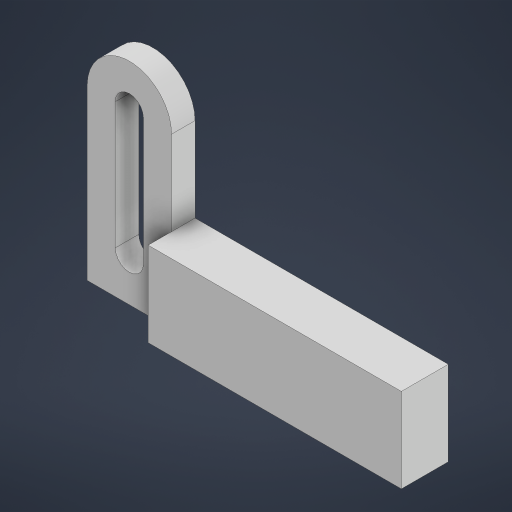
# Autodesk Inventor part: Slider2
Saved by Autodesk Inventor 2024 (Build 280153000, 153)
## iProperties
Created: 2024-02-06
Part Number: Slider2
Material: Generic
Document SubType Name: Modeling
Designer: calvi
Density: 1 g/cm^3
Appearance: Default
Author: calvi
Autodesk Inventor part; units mm, degrees
ref_plane "YZ Plane" through (0, 0, 0) normal (1, 0, 0) x (0, 1, 0)
ref_plane "XZ Plane" through (0, 0, 0) normal (0, 1, 0) x (-1, 0, 0)
ref_plane "XY Plane" through (0, 0, 0) normal (0, 0, 1) x (1, 0, 0)
sketch "Sketch1" plane through (0, 0, 0) normal (0, 0, 1) x (1, 0, 0)
  line L0 (0, 0) -> (22.86, 0)
  line L1 (22.86, 0) -> (22.86, 91.44)
  line L2 (22.86, 91.44) -> (0, 91.44)
  line L3 (0, 91.44) -> (0, 0)
  line L4 (22.86, 57.15) -> (91.44, 57.15)
  line L5 (91.44, 57.15) -> (91.44, 34.29)
  line L6 (91.44, 34.29) -> (22.86, 34.29)
  line L7 (22.86, 34.29) -> (22.86, 57.15)
  line L8 (11.43, 80.01) -> (11.43, 11.43) construction
  line L9 (7.62, 80.01) -> (7.62, 11.43)
  line L10 (15.24, 11.43) -> (15.24, 80.01)
  arc A0 (15.24, 80.01) -> (7.62, 80.01) centre (11.43, 80.01) ccw
  arc A1 (7.62, 11.43) -> (15.24, 11.43) centre (11.43, 11.43) ccw
  arc A2 (22.86, 80.01) -> (0, 80.01) centre (11.43, 80.01) ccw
  arc A3 (0, 11.43) -> (22.86, 11.43) centre (11.43, 11.43) ccw
  point P0 (11.43, 45.72)
  point P1 (-17.5605, -7.6237)
  dimension "d0" = 22.86
  dimension "d1" = 91.44
  dimension "d2" = 68.58
  dimension "d3" = 22.86
  dimension "d4" = 34.29
  dimension "d5" = 68.58
  dimension "d6" = 7.62
  dimension "d7" = 11.43
  dimension "d8" = 11.43
  dimension "d9" = 0
  dimension "d10" = 0
  constraints: 24 end point, 8 point on circle, 6 tangent, 5 parallel, 5 point on line, 4 centre point, 2 coincident, 2 horizontal, 2 perpendicular, 1 midpoint, 1 vertical
  measures "d0" distance of L2.end L1.end
  measures "d1" distance of L1.end L0.end
  measures "d2" distance of L5.end L6.end
  measures "d3" distance of L4.end L5.end
  measures "d4" distance between parallel lines of L4 L2
  measures "d5" distance of L8.start L8.end
  measures "d6" diameter of A1
  measures "d7" distance from line of L2 L8.start
  measures "d8" distance from line of L3 L8.start
  measures "d9" distance of point (0, 0) L0.start
  measures "d10" distance of point (0, 0) L0.start
extrude "Extrusion1" add sketch "Sketch1" along normal blind 12.7 contours A3 L3 A2 L1 | L1 L4 L5 L6
sketch "Sketch2" plane through (0, 0, 12.7) normal (0, 0, 1) x (1, 0, 0)
  line L0 (22.86, 0) -> (0, 0)
  line L1 (0, 0) -> (0, 91.44)
  line L2 (0, 91.44) -> (22.86, 91.44)
  line L3 (22.86, 91.44) -> (22.86, 0)
  line L4 (0, 80.01) -> (0, 11.43) projected
  line L5 (22.86, 57.15) -> (22.86, 80.01) projected
  arc A0 (22.86, 80.01) -> (0, 80.01) centre (11.43, 80.01) ccw projected
  arc A1 (0, 11.43) -> (22.86, 11.43) centre (11.43, 11.43) ccw projected
  point P0 (0, 0)
  point P1 (0, 11.43)
  dimension "d13" = 0
  dimension "d14" = 0
  constraints: 8 end point, 2 parallel, 2 tangent, 1 horizontal, 1 perpendicular
  measures "d13" distance between parallel lines of L4 L1
  measures "d14" distance between parallel lines of L5 L3
extrude "Extrusion2" cut sketch "Sketch2" against normal blind 6.35 contours A1 L1 A0 L3
sketch "Sketch3" plane through (0, 0, 6.35) normal (0, 0, 1) x (1, 0, 0)
  line L0 (22.86, 34.29) -> (91.44, 34.29) projected
  line L1 (22.86, 34.29) -> (0, 34.29)
  line L2 (0, 34.29) -> (0, 0)
  line L3 (0, 0) -> (22.86, 0)
  line L4 (22.86, 0) -> (22.86, 34.29)
  line L5 (0, 11.43) -> (0, 80.01) projected
  arc A0 (0, 11.43) -> (22.86, 11.43) centre (11.43, 11.43) ccw projected
  point P0 (0, 0)
  dimension "d17" = 0
  constraints: 8 end point, 2 parallel, 1 horizontal, 1 perpendicular, 1 tangent
  measures "d17" distance between parallel lines of L5 L2
extrude "Extrusion3" cut sketch "Sketch3" against normal blind 107.95 contours L4 A0 L2 L1
sketch "Sketch4" plane through (0, 0, 6.35) normal (0, 0, 1) x (1, 0, 0)
  line L0 (22.86, 34.29) -> (0, 34.29)
  line L1 (0, 34.29) -> (0, 41.91)
  line L2 (22.86, 41.91) -> (22.86, 34.29)
  arc A0 (7.62, 45.72) -> (15.24, 45.72) centre (11.43, 45.72) ccw
  line L3 (15.24, 34.29) -> (15.24, 80.01) projected
  line L4 (15.24, 41.91) -> (15.24, 45.72)
  line L5 (7.62, 80.01) -> (7.62, 34.29) projected
  line L6 (7.62, 41.91) -> (7.62, 45.72)
  line L7 (0, 41.91) -> (7.62, 41.91)
  line L8 (15.24, 41.91) -> (22.86, 41.91)
  point P0 (0, 0)
  dimension "d20" = 22.86
  dimension "d21" = 7.62
  dimension "d22" = 7.62
  constraints: 14 end point, 4 point on line, 3 parallel, 3 tangent, 2 point on circle, 1 centre point, 1 horizontal, 1 perpendicular
  measures "d20" distance of L1.end L2.start
  measures "d21" distance of L0.end L1.end
  measures "d22" diameter of A0
extrude "Extrusion4" add sketch "Sketch4" against normal blind 6.35 contours L0 L5 A0 L3
body "Solid1"
